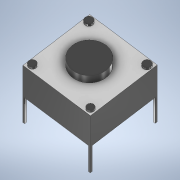
# Autodesk Inventor part: switch
Saved by Autodesk Inventor 2022 (Build 260153070, 153G)
## iProperties
Created: 2021-07-13
Part Number: switch
Material: Generic
Document SubType Name: Modeling
Designer: sachin
Density: 1 g/cm^3
Appearance: Default
Author: sachin
Autodesk Inventor part; units mm, degrees
ref_plane "YZ Plane" through (0, 0, 0) normal (1, 0, 0) x (0, 1, 0)
ref_plane "XZ Plane" through (0, 0, 0) normal (0, 1, 0) x (-1, 0, 0)
ref_plane "XY Plane" through (0, 0, 0) normal (0, 0, 1) x (1, 0, 0)
sketch "Sketch1" plane through (0, 0, 0) normal (0, 1, 0) x (-1, 0, 0)
  line L0 (15.3914, 31.136) -> (0.1514, 31.136)
  line L1 (0.1514, 31.136) -> (0.1514, 15.896)
  line L2 (0.1514, 15.896) -> (15.3914, 15.896)
  line L3 (15.3914, 15.896) -> (15.3914, 31.136)
  point P0 (0, 0)
  dimension "d0" = 15.24
  dimension "d1" = 15.24
  constraints: 8 end point, 2 parallel, 1 horizontal, 1 perpendicular
  measures "d0" distance of L2.end L0.start
  measures "d1" distance of L1.end L2.end
extrude "Extrusion1" add sketch "Sketch1" along normal blind 7.62
sketch "Sketch2" plane through (0, 0, 0) normal (0, -1, 0) x (1, 0, 0)
  circle A0 centre (-7.8533, 23.6101) radius 3.7937
  point P0 (0, 0)
  constraints: 1 centre point
extrude "Extrusion2" add sketch "Sketch2" along normal blind 1.778
sketch "Sketch3" plane through (0, 0, 0) normal (0, -1, 0) x (1, 0, 0)
  circle A0 centre (-1.4346, 30.0524) radius 0.8632
  circle A1 centre (-1.4346, 16.9205) radius 0.8792
  circle A2 centre (-14.354, 30.0524) radius 0.8098
  circle A3 centre (-14.354, 16.9205) radius 0.7609
  point P0 (0, 0)
  constraints: 4 centre point
extrude "Extrusion3" add sketch "Sketch3" along normal blind 0.508
sketch "Sketch4" plane through (0, 7.62, 0) normal (0, 1, 0) x (1, 0, 0)
  line L0 (-15.3914, -15.896) -> (-15.3914, -31.136) projected
  line L1 (-15.3914, -31.136) -> (-14.9868, -31.136)
  line L2 (-14.9868, -31.136) -> (-14.9868, -30.723)
  line L3 (-14.9868, -30.723) -> (-15.3914, -30.723)
  line L4 (-15.3914, -30.723) -> (-15.3914, -31.136)
  line L5 (-0.1514, -15.896) -> (-15.3914, -15.896) projected
  line L6 (-15.3914, -15.896) -> (-14.9868, -15.896)
  line L7 (-14.9868, -15.896) -> (-14.9868, -16.2998)
  line L8 (-14.9868, -16.2998) -> (-15.3914, -16.2998)
  line L9 (-15.3914, -16.2998) -> (-15.3914, -15.896)
  line L10 (-0.1514, -15.896) -> (-0.5623, -15.896)
  line L11 (-0.5623, -15.896) -> (-0.5623, -16.3119)
  line L12 (-0.5623, -16.3119) -> (-0.1514, -16.3119)
  line L13 (-0.1514, -16.3119) -> (-0.1514, -15.896)
  line L14 (-15.3914, -31.136) -> (-0.1514, -31.136) projected
  line L15 (-0.1514, -31.136) -> (-0.5623, -31.136)
  line L16 (-0.5623, -31.136) -> (-0.5623, -30.723)
  line L17 (-0.5623, -30.723) -> (-0.1514, -30.723)
  line L18 (-0.1514, -30.723) -> (-0.1514, -31.136)
  point P0 (0, 0)
  constraints: 32 end point, 8 parallel, 4 horizontal, 4 perpendicular, 3 point on line
extrude "Extrusion4" add sketch "Sketch4" along normal blind 6.35
body "Solid1"
